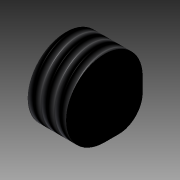
# Autodesk Inventor part: Gewindestift DIN 913 - M4x3_
Saved by Autodesk Inventor 2014 SP2 (Build 180246200, 246)
## iProperties
Created: 2018-08-04
Part Number: Gewindestift DIN 913 - M4x3_
Material: Generic
Catalog Web Link: www.cadenas.de
Description: DIN 913_-Gewindestift mit Innensechskant und Kegelkuppe
Vendor: MISUMI
Document SubType Name: Modeling
Designer: psadmin
Manufacturer: MISUMI
Mass: 0.0287636 g
Surface Area: 0.64306 cm^2
Volume: 0.0287636 cm^3
Density: 1 g/cm^3
Appearance: PSOLRGB-0-0-0
Category: PARTsolutions
Company: MISUMI
Title: Gewindestift DIN 913 - M4x3_
Author: Cadenas PARTsolutions
Comments: Gewindestift mit Innensechskant und Kegelkuppe
PSOL_IDENT_0: {$CADENAS_DATA\23d-libs\misumi\metric\51_timing_pulleys\din_913_1.prj},201 {VTYP=3D},{NB=Gewindestif
PSOL_IDENT_1: t DIN 913 - M4x3_},{LINA=Gewindestift DIN 913 - M4x3_},{NN=DIN 913_},{DATE=30.03.2018 07:25:55},{GEO
PSOL_IDENT_2: MDATE=17.02.2014 00:00:00},{VERSION=v1},{LINEID=320},{WBVAR=},{WBNUMERIC=}  {NB=Gewindestift DIN 913
PSOL_IDENT_3: - M4x3_},{LINA=Gewindestift DIN 913 - M4x3_},{KT=X},{IDNR=},{NENN=M4x3},{D=4.000},{D3=3.141},{P=0.7
PSOL_IDENT_4: 00},{L=3.000},{DP=2.500},{S=2.000},{T=1.500}
NN: DIN 913_
NT: Hexagon socket set screw with flat point
NB: Gewindestift DIN 913 - M4x3_
NBSYN: Gewindestift DIN 913 - $NENN._
LINA: Gewindestift DIN 913 - M4x3_
ROWDESC: M4x3
D: 4
D3: 3.141
P: 0.7
L: 3
DP: 2.5
S: 2
T: 1.5
SUPPLIER: MISUMI
ARTICLENO: Gewindestift DIN 913 - M4x3_
BOMINFO: Gewindestift DIN 913 - M4x3_
CREATOR: CADENAS GmbH
Autodesk Inventor part; units mm, degrees
sketch "Sketch_1" plane through (0, 0, 0) normal (0, 0, 1) x (1, 0, 0)
  line L0 (0.6667, 0) -> (3, 0)
  line L1 (3, 0) -> (3, -1.25)
  line L2 (3, -1.25) -> (2.25, -2)
  line L3 (2.25, -2) -> (0.248, -2)
  line L4 (0.248, -2) -> (0, -1.5705)
  line L5 (0, -1.5705) -> (0, -1.1547)
  line L6 (0, -1.1547) -> (0.6667, 0)
  line L7 (0.6667, 0) -> (3, 0)
  constraints: 16 end point
revolve "Revolution1" add sketch "Sketch_1" angle 360 about axis through (0.6667, 0, 0) along (1, 0, 0)
thread "Thread1" size "M4x0.7" class "6g" standard "ISO Metric profile" full length
sketch "Sketch_2" plane through (0, 0, 0) normal (1, 0, 0) x (0, 1, 0)
  line L0 (0, 1.1547) -> (-1, 0.5774)
  line L1 (-1, 0.5774) -> (-1, -0.5774)
  line L2 (-1, -0.5774) -> (0, -1.1547)
  line L3 (0, -1.1547) -> (1, -0.5774)
  line L4 (1, -0.5774) -> (1, 0.5774)
  line L5 (1, 0.5774) -> (0, 1.1547)
  constraints: 12 end point
extrude "Extrusion1" cut sketch "Sketch_2" along normal blind 1.5
ref_plane "IP1_XY" through (0, 0, 0) normal (1, 0, 0) x (0, 0, -1)
ref_plane "IP1_YZ" through (0, 0, 0) normal (0, 0, -1) x (0, 1, 0)
ref_plane "IP1_ZX" through (0, 0, 0) normal (0, 1, 0) x (1, 0, 0)
ref_plane "IP2_XY" through (3, 0, 0) normal (1, 0, 0) x (0, 0, -1)
ref_plane "IP2_YZ" through (3, 0, 0) normal (0, 0, -1) x (0, 1, 0)
ref_plane "IP2_ZX" through (3, 0, 0) normal (0, 1, 0) x (1, 0, 0)
body "Solid1"
